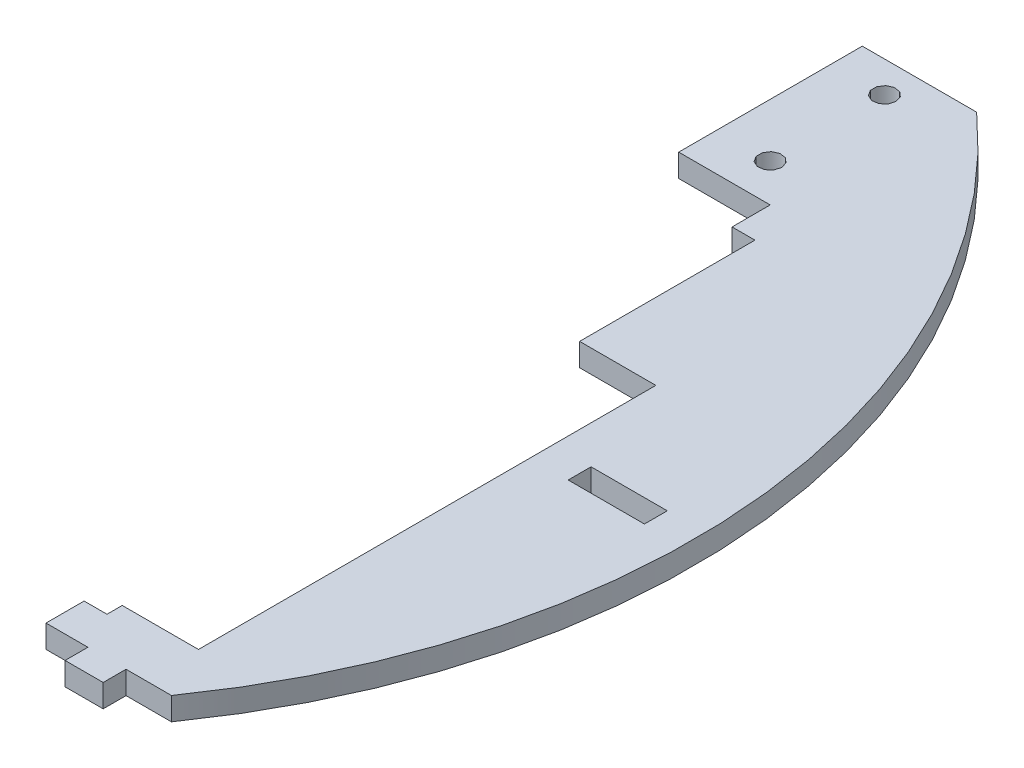
# Autodesk Inventor part: Out side rib
Saved by Autodesk Inventor 2015 (Build 190159000, 159)
## iProperties
Created: 2014-11-13
Part Number: Out side rib
Material: Generic
Document SubType Name: Modeling
Designer: karl
Density: 1 g/cm^3
Appearance: Default
Author: karl
Autodesk Inventor part; units mm, degrees
ref_plane "YZ Plane" through (0, 0, 0) normal (1, 0, 0) x (0, 1, 0)
ref_plane "XZ Plane" through (0, 0, 0) normal (0, 1, 0) x (-1, 0, 0)
ref_plane "XY Plane" through (0, 0, 0) normal (0, 0, 1) x (1, 0, 0)
sketch "Sketch1" plane through (0, 0, 0) normal (0, 1, 0) x (-1, 0, 0)
  circle A0 centre (0, 0) radius 90
  line L0 (73.4575, 52) -> (-73.4575, 52)
  dimension "d0" = 180
  dimension "d1" = 52
  constraints: 2 end point, 2 point on circle, 1 centre point, 1 coincident, 1 horizontal
  measures "d0" diameter of A0
  measures "d1" distance from line of point (0, 0) L0
extrude "Extrusion1" add sketch "Sketch1" along normal blind 3 contours A0 L0 picked at (17.1608, -0.9679)
sketch "Sketch2" plane through (0, 3, 0) normal (0, 1, 0) x (1, 0, 0)
  line L0 (-73.4575, -52) -> (73.4575, -52) projected
  line L1 (60, -52) -> (-90, -52)
  line L2 (-90, -52) -> (-90, 90)
  line L3 (-90, 90) -> (60, 90)
  line L4 (60, 90) -> (60, -52)
  arc A0 (73.4575, -52) -> (-73.4575, -52) centre (0, 0) ccw projected
  dimension "d4" = 60
  constraints: 8 end point, 2 parallel, 2 tangent, 1 horizontal, 1 perpendicular, 1 point on line
  measures "d4" distance from line of L4 point (0, 0)
extrude "Extrusion2" cut sketch "Sketch2" against normal blind 3 contours A0 L4 L0 | L1 L2 A0 | L2 L3 A0 | A0 L3 L4 picked at (-22.3183, 24.985)
sketch "Sketch3" plane through (0, 3, 0) normal (0, 1, 0) x (1, 0, 0)
  line L0 (60, 67.082) -> (45, 67.082)
  line L1 (45, 67.082) -> (45, 43)
  line L2 (45, 43) -> (60, 43)
  line L3 (60, 43) -> (60, 67.082)
  line L4 (60, -52) -> (73.4575, -52) projected
  line L5 (60, -52) -> (57, -52)
  line L6 (57, -52) -> (57, -47)
  line L7 (57, -47) -> (60, -47)
  line L8 (60, -47) -> (60, -52)
  point P0 (0, 0)
  dimension "d7" = 15
  dimension "d8" = 95
  dimension "d9" = 3
  dimension "d10" = 5
  constraints: 16 end point, 4 parallel, 2 horizontal, 2 perpendicular
  measures "d7" distance of L2.end L1.end
  measures "d8" distance between parallel lines of L4 L2
  measures "d9" distance of L6.end L7.end
  measures "d10" distance of L5.end L6.end
extrude "Extrusion3" add sketch "Sketch3" against normal blind 3
sketch "Sketch4" plane through (0, 3, 0) normal (0, 1, 0) x (1, 0, 0)
  line L0 (60, -47) -> (60, 43) projected
  line L1 (60, -45) -> (70, -45)
  line L2 (70, -45) -> (70, 15)
  line L3 (70, 15) -> (60, 15)
  line L4 (60, 15) -> (60, -45)
  line L5 (57, -52) -> (73.4575, -52) projected
  point P0 (0, 0)
  dimension "d13" = 10
  dimension "d14" = 60
  dimension "d15" = 7
  constraints: 8 end point, 2 parallel, 1 horizontal, 1 perpendicular, 1 point on line
  measures "d13" distance of L3.end L2.end
  measures "d14" distance of L2.end L1.end
  measures "d15" distance between parallel lines of L5 L1
extrude "Extrusion4" cut sketch "Sketch4" against normal blind 3
sketch "Sketch5" plane through (0, 3, 0) normal (0, 1, 0) x (1, 0, 0)
  line L0 (75, -1.5) -> (85, -1.5)
  line L1 (85, -1.5) -> (85, 1.5)
  line L2 (85, 1.5) -> (75, 1.5)
  line L3 (75, 1.5) -> (75, -1.5)
  line L4 (70, -45) -> (70, 15) projected
  point P0 (0, 0)
  point P1 (75, 0)
  dimension "d18" = 10
  dimension "d19" = 3
  dimension "d20" = 5
  constraints: 8 end point, 2 parallel, 1 horizontal, 1 horizontal alignment, 1 midpoint, 1 perpendicular
  measures "d18" distance of L2.end L1.end
  measures "d19" distance of L1.end L0.end
  measures "d20" distance between parallel lines of L4 L3
extrude "Extrusion5" cut sketch "Sketch5" against normal blind 3
sketch "Sketch6" plane through (0, 3, 0) normal (0, 1, 0) x (1, 0, 0)
  circle A0 centre (52, 48) radius 1.5
  circle A1 centre (52, 63) radius 1.5
  line L0 (60, 43) -> (60, 15) projected
  line L1 (45, 43) -> (60, 43) projected
  point P0 (0, 0)
  dimension "d23" = 3
  dimension "d24" = 3
  dimension "d25" = 15
  dimension "d26" = 8
  dimension "d27" = 5
  constraints: 2 centre point, 1 vertical alignment
  measures "d23" diameter of A0
  measures "d24" diameter of A1
  measures "d25" distance of A1.centre A0.centre
  measures "d26" distance from line of L0 A0.centre
  measures "d27" distance from line of L1 A0.centre
extrude "Extrusion6" cut sketch "Sketch6" against normal blind 3
sketch "Sketch7" plane through (0, 3, 0) normal (0, 1, 0) x (1, 0, 0)
  line L0 (60, 43) -> (57, 43)
  line L1 (57, 43) -> (57, 38)
  line L2 (57, 38) -> (60, 38)
  line L3 (60, 38) -> (60, 43)
  point P0 (0, 0)
  dimension "d30" = 3
  dimension "d31" = 5
  constraints: 8 end point, 2 parallel, 1 horizontal, 1 perpendicular
  measures "d30" distance of L2.end L1.end
  measures "d31" distance of L1.end L0.end
extrude "Extrusion7" add sketch "Sketch7" against normal blind 3
sketch "Sketch8" plane through (0, 3, 0) normal (0, 1, 0) x (1, 0, 0)
  line L0 (57, -52) -> (73.4575, -52) projected
  line L1 (62.5, -52) -> (67.5, -52)
  line L2 (67.5, -52) -> (67.5, -55)
  line L3 (67.5, -55) -> (62.5, -55)
  line L4 (62.5, -55) -> (62.5, -52)
  line L5 (60, -45) -> (60, -47) projected
  point P0 (0, 0)
  dimension "d34" = 5
  dimension "d35" = 3
  dimension "d36" = 2.5
  constraints: 8 end point, 2 parallel, 1 horizontal, 1 perpendicular, 1 point on line
  measures "d34" distance of L2.end L3.end
  measures "d35" distance of L1.end L2.end
  measures "d36" distance between parallel lines of L5 L4
extrude "Extrusion8" add sketch "Sketch8" against normal blind 3
body "Solid1"
